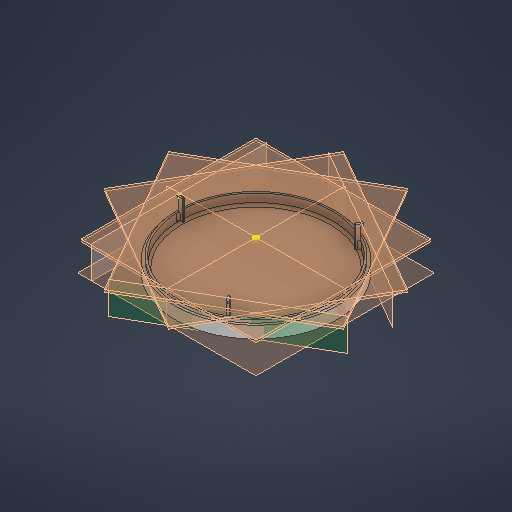
# Autodesk Inventor part: plate
Saved by Autodesk Inventor 2026 (Build 300175050, 175E)
## iProperties
Created: 2025-07-28
Part Number: plate
Material: Generic
Document SubType Name: Modeling
Designer: bruno
Density: 1 g/cm^3
Appearance: Default
Author: bruno
Autodesk Inventor part; units mm, degrees
sketch "Sketch1" plane through (0, 0, 0) normal (0, 1, 0) x (-1, 0, 0)
  circle A0 centre (0, 0) radius 54
  dimension "d0" = 108
  constraints: 1 centre point, 1 coincident
  measures "d0" diameter of A0
extrude "Extrusion1" add sketch "Sketch1" along normal blind 10
shell "Shell1" thickness 3 removed faces 1 at (7.7603, 10, 10.4365)
sketch "Sketch2" plane through (0, 10, 0) normal (0, 1, 0) x (1, 0, 0)
  circle A0 centre (0, 0) radius 54 projected
  circle A1 centre (0, 0) radius 51 projected
  circle A2 centre (0, 0) radius 54 projected
  circle A3 centre (0, 0) radius 52.3
  dimension "d4" = 1.3
  constraints: 1 centre point
  measures "d4" radial gap between concentric circles of A1 A3
extrude "Extrusion2" cut sketch "Sketch2" against normal blind 2 contours A0
fillet "Fillet1" radius 1.5 1 edges at (51, 3, 0)
ref_plane "Work Plane1" through (0, 18, 0) normal (0, 1, 0) x (-1, 0, 0)
sketch "Sketch3" plane through (0, 18, 0) normal (0, 1, 0) x (-1, 0, 0)
  circle A0 centre (0, 0) radius 52.3 projected
  circle A1 centre (0, 0) radius 51 projected
  line L0 (-75.6, 0) -> (75.6, 0) projected
  circle A2 centre (52.3, 0) radius 0.75
  line L1 (52.2946, 0.75) -> (0, 0)
  line L2 (0, 0) -> (52.2946, -0.75)
  point P0 (50.9948, 0.7313)
  point P1 (50.9948, -0.7313)
  dimension "d9" = 1.5
  constraints: 5 point on circle, 4 end point, 1 centre point, 1 point on line
  measures "d9" diameter of A2
extrude "Extrusion3" add sketch "Sketch3" along normal blind 1.5 contours A2 L0 A1 L1 | L0 A2 A0 | A0 A2 L0 | L2 A1 L0 A2 picked at (52.0743, 0.1913) picked at (52.0743, -0.1913)
fillet "Fillet2" radius 0.5 2 edges at (-52.2946, 18.75, -0.75) (-52.2946, 18.75, 0.75)
sketch "Sketch4" plane through (0, 18, 0) normal (0, 1, 0) x (-1, 0, 0)
  arc A0 (50.9948, -0.7313) -> (50.9948, 0.7313) centre (0, 0) ccw projected
ref_plane "Work Plane2" through (0, 19.5, 0) normal (0, 1, 0) x (-1, 0, 0)
sketch "Sketch5" plane through (0, 19.5, 0) normal (0, 1, 0) x (-1, 0, 0)
  arc A0 (50.9948, -0.7313) -> (50.9948, 0.7313) centre (0, 0) ccw projected
sketch "Sketch6" plane through (0, 19.5, 0) normal (0, 1, 0) x (-1, 0, 0)
  line L0 (51.7923, 0.7428) -> (50.9948, 0.7313) projected
  line L1 (50.9948, 0.7313) -> (0, 0)
  arc A0 (50.9948, -0.7313) -> (50.9948, 0.7313) centre (0, 0) ccw projected
  line L2 (0, 0) -> (50.9948, -0.7313)
  circle A1 centre (0, 0) radius 48
  point P0 (47.9951, 0.6883)
  point P1 (47.9951, -0.6883)
  dimension "d15" = 96
  constraints: 4 end point, 1 centre point, 1 coincident, 1 collinear
  measures "d15" diameter of A1
extrude "Extrusion4" add sketch "Sketch6" against normal blind 14.5 contours A0 L2 A1 L1
fillet "Fillet3" radius 0.5 2 edges at (-47.9951, 12.25, -0.6883) (-47.9951, 12.25, 0.6883)
fillet "Fillet4" radius 1.5 2 edges at (-50.9948, 7.5, -0.7313) (-50.9948, 7.5, 0.7313)
ref_plane "Work Plane5" through (-51, 0, 0) normal (1, 0, 0) x (0, 1, 0)
sketch "Sketch7" plane through (-51, 0, 0) normal (1, 0, 0) x (0, 1, 0)
  line L0 (18, -0.7428) -> (18, -0.2452) projected
  line L1 (18, 0.7313) -> (10, 0.7313) projected
  line L2 (18, -0.7428) -> (10, -0.7428)
  line L3 (10, -0.7428) -> (10, 0.7313)
  line L4 (10, 0.7313) -> (18, 0.7313)
  line L5 (18, 0.7313) -> (18, -0.7428)
  point P0 (0, 0)
  point P1 (18, -0.2452)
  constraints: 8 end point, 2 parallel, 1 perpendicular
extrude "Extrusion5" cut sketch "Sketch7" along normal blind 0.2
pattern_circular "Circular Pattern2" count 3 over 360 about axis through (0, -10, 0) along (0, 1, 0) of "Extrusion3", "Fillet2", "Extrusion4", "Fillet3", "Fillet4", "Extrusion5"
fillet "Fillet5" radius 0.5 8 edges at (-50.1423, 19.5, 0.7191) (-52.1496, 19.5, 0.5997) (-52.3, 19.5, 0) (-52.1496, 19.5, -0.5997) (-50.1423, 19.5, -0.7191) (-48.1428, 19.5, -0.5458) (-48, 19.5, 0) (-48.1428, 19.5, 0.5458)
fillet "Fillet6" radius 0.5 7 edges at (-50.5421, 5, 1.1804) (-48.1428, 5, 0.5458) (-48, 5, 0) (-48.1428, 5, -0.5458) (-48.9823, 5, -0.7025) (-50.5421, 5, -1.1804) (-48.9823, 5, 0.7025)
ref_plane "Work Plane6" through (0, 18, 0) normal (0, 1, 0) x (0.5, 0, 0.8660254)
ref_plane "Work Plane7" through (0, 18, 0) normal (0, 1, 0) x (0.5, 0, -0.8660254)
ref_plane "Work Plane8" through (25.5, 0, 44.1673) normal (-0.5, 0, -0.8660254) x (0, 1, 0)
ref_plane "Work Plane9" through (25.5, 0, -44.1673) normal (-0.5, 0, 0.8660254) x (0, 1, 0)
ref_plane "Work Plane10" through (0, 19.5, 0) normal (0, 1, 0) x (0.5, 0, 0.8660254)
ref_plane "Work Plane11" through (0, 19.5, 0) normal (0, 1, 0) x (0.5, 0, -0.8660254)
body "Solid1"
